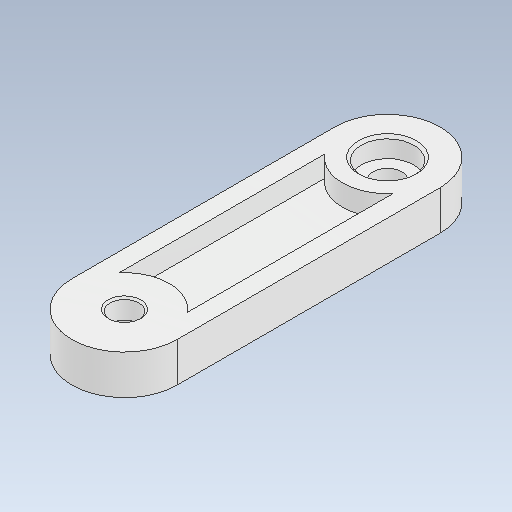
# Autodesk Inventor part: ramię_korby
Saved by Autodesk Inventor 2020 (Build 240168000, 168)
## iProperties
Created: 2020-08-09
Part Number: ramię_korby
Material: ABS Plastic
Document SubType Name: Modeling
Designer: Hesekiel
Density: 1.06 g/cm^3
Appearance: Smooth - White
Mass: 61.6212 g
Surface Area: 181.039 cm^2
Volume: 58.1332 cm^3
Author: Hesekiel
Autodesk Inventor part; units mm, degrees
ref_plane "YZ Plane" through (0, 0, 0) normal (1, 0, 0) x (0, 1, 0)
ref_plane "XZ Plane" through (0, 0, 0) normal (0, 1, 0) x (-1, 0, 0)
ref_plane "XY Plane" through (0, 0, 0) normal (0, 0, 1) x (1, 0, 0)
sketch "Sketch1" plane through (0, 0, 0) normal (0, 1, 0) x (-1, 0, 0)
  circle A0 centre (0, 0) radius 10
  circle A1 centre (0, 0) radius 20
  line L0 (0, 0) -> (0, -100)
  circle A2 centre (0, -100) radius 10
  circle A3 centre (0, -100) radius 20
  line L1 (0, -100) -> (20, -100)
  line L2 (20, -100) -> (20, 0)
  line L3 (20, 0) -> (0, 0)
  line L4 (0, 0) -> (0, -100)
  line L5 (0, -100) -> (-20, -100)
  line L6 (-20, -100) -> (-20, 0)
  line L7 (-20, 0) -> (0, 0)
  line L8 (0, 0) -> (0, -100)
  point P0 (20, -100)
  dimension "d0" = 20
  dimension "d4" = 40
  dimension "d23" = 20
  dimension "d24" = 40
  constraints: 18 end point, 4 centre point, 4 coincident, 4 parallel, 2 horizontal, 2 perpendicular, 2 point on circle, 1 vertical
  measures "d0" diameter of A0
  measures "d4" diameter of A1
  measures "d23" diameter of A2
  measures "d24" diameter of A3
extrude "Extrusion1" add sketch "Sketch1" along normal blind 15 contours L3 A1 L0 A0 | A0 L7 A1 L3 | A0 L0 A1 L7 | L2 A3 L0 A1 | A1 L0 A3 L6 | L1 A2 L0 A3 | A3 L5 A2 L1 | A3 L0 A2 L5
shell "Shell2" thickness 7 removed faces 1 at (-15.2269, 15, -36.0766)
sketch "Sketch8" plane through (0, 15, 0) normal (0, 1, 0) x (1, 0, 0)
  line L0 (-13, 10.9545) -> (-13, 89.0455) projected
  arc A0 (-13, 89.0455) -> (13, 89.0455) centre (0, 100) ccw projected
  line L1 (13, 89.0455) -> (13, 10.9545) projected
  arc A1 (13, 10.9545) -> (-13, 10.9545) centre (0, 0) ccw projected
  arc A2 (-20, 0) -> (20, 0) centre (0, 0) ccw projected
  line L2 (20, 0) -> (20, 100) projected
  arc A3 (20, 100) -> (-20, 100) centre (0, 100) ccw projected
  line L3 (-20, 100) -> (-20, 0) projected
  circle A4 centre (0, 0) radius 10 projected
  circle A5 centre (0, 100) radius 10 projected
  circle A6 centre (0, 0) radius 5.5
  circle A7 centre (0, 100) radius 5.5
  dimension "d26" = 11
  dimension "d27" = 11
  constraints: 2 centre point, 2 coincident
  measures "d26" diameter of A6
  measures "d27" diameter of A7
extrude "Extrusion8" add sketch "Sketch8" against normal blind 7.5 contours A4
sketch "Sketch9" plane through (0, 0, 0) normal (0, -1, 0) x (1, 0, 0)
  arc A0 (20, 0) -> (-20, 0) centre (0, 0) ccw projected
  line L0 (-20, -100) -> (-20, 0) projected
  arc A1 (-20, -100) -> (20, -100) centre (0, -100) ccw projected
  line L1 (20, 0) -> (20, -100) projected
  circle A2 centre (0, 0) radius 10 projected
  circle A3 centre (0, -100) radius 10 projected
  circle A4 centre (0, -100) radius 5.5
  dimension "d30" = 11
  constraints: 1 centre point, 1 coincident
  measures "d30" diameter of A4
extrude "Extrusion9" add sketch "Sketch9" against normal blind 7.5 contours A3
chamfer "Chamfer1" distance 1 angle 45 2 edges at (10, 15, -100) (10, 0, 0)
chamfer "Chamfer2" distance 0.7 angle 45 2 edges at (-5.5, 15, 0) (-5.5, 0, -100)
body "Solid1"
